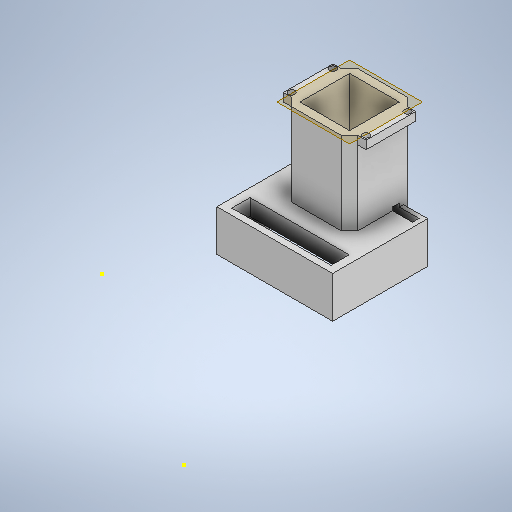
# Autodesk Inventor part: Soporte camara
Saved by Autodesk Inventor 2025 (Build 290162000, 162)
## iProperties
Created: 2025-02-01
Part Number: Soporte camara
Material: Genérico
Document SubType Name: Modeling
Designer: Jorge
Density: 1 g/cm^3
Appearance: Valor por defecto
Author: Jorge
Autodesk Inventor part; units mm, degrees
ref_plane "YZ Plane" through (0, 0, 0) normal (1, 0, 0) x (0, 1, 0)
sketch "Boceto1" plane through (0, 0, 0) normal (0, 1, 0) x (-1, 0, 0)
  line L0 (0, 0) -> (0, -154)
  line L1 (35, -185) -> (95, -185)
  line L2 (130, -154) -> (130, 0)
  line L3 (130, 0) -> (0, 0)
  line L4 (0, 0) -> (0, -154) construction
  line L5 (65, -185) -> (95, -185) construction
  line L6 (95, -185) -> (95, -206.4869) construction
  line L7 (95, -206.4869) -> (35, -206.4869) construction
  line L8 (35, -206.4869) -> (35, -185) construction
  line L9 (0, -154) -> (35, -185)
  line L10 (95, -185) -> (130, -154)
  line L11 (61.4516, 0) -> (61.4516, -5) construction
  line L12 (130, -81.3037) -> (125, -81.3037) construction
  line L13 (0, -85.0807) -> (5, -85.0807) construction
  line L14 (125, -5) -> (5, -5)
  line L15 (5, -5) -> (5, -148.3548)
  line L16 (125, -148.3548) -> (125, -5)
  line L17 (112.5, -169.5) -> (109.1848, -165.7571) construction
  line L18 (65, -185) -> (65, -180) construction
  line L19 (17.5, -169.5) -> (20.8152, -165.7571) construction
  line L20 (20.8152, -165.7571) -> (5, -151.7493)
  line L21 (20.8152, -165.7571) -> (36.8959, -180)
  line L22 (36.8959, -180) -> (93.1041, -180)
  line L23 (93.1041, -180) -> (125, -151.7493)
  line L24 (125, -151.7493) -> (125, -148.3548)
  line L25 (5, -148.3548) -> (5, -151.7493)
  dimension "d2" = 154
  dimension "d3" = 30
  dimension "d4" = 60
  dimension "d5" = 5
  dimension "d6" = 5
  dimension "d7" = 5
  dimension "d8" = 5
  dimension "d9" = 5
  dimension "d10" = 5
  constraints: 52 end point, 9 perpendicular, 4 horizontal, 3 midpoint, 3 point on line, 3 vertical, 2 parallel
  measures "d2" distance of L0.end L0.start
  measures "d3" distance of L1.end L5.start
  measures "d4" distance of L6.end L7.end
  measures "d5" distance of L11.start L11.end
  measures "d6" distance of L12.start L12.end
  measures "d7" distance of L13.start L13.end
  measures "d8" distance of L17.start L17.end
  measures "d9" distance of L5.start L18.end
  measures "d10" distance of L19.start L19.end
extrude "Extrusión1" add sketch "Boceto1" along normal blind 3 contours L16 L24 L23 L22 L21 L20 L25 L15 L14
extrude "Extrusión2" add sketch "Boceto1" along normal blind 35
ref_plane "Plano de trabajo1" through (0, 20, 0) normal (0, 1, 0) x (-1, 0, 0)
sketch "Boceto2" plane through (0, 20, 0) normal (0, 1, 0) x (-1, 0, 0)
  line L0 (0, 0) -> (0, -154) construction
  line L1 (0, 0) -> (0, -26.749) construction
  line L2 (130, -154) -> (130, 0) construction
  line L3 (125, -151.7493) -> (93.1041, -180) construction
  line L4 (125, -151.7493) -> (5, -151.7493) construction
  line L5 (65, -151.7493) -> (65, -26.749) construction
  line L6 (125, -89.2492) -> (5, -89.2492) construction
  line L7 (5, -151.7493) -> (5, -5) construction
  line L8 (125, -26.749) -> (125, -31.749) construction
  line L9 (125, -31.749) -> (120, -31.749) construction
  line L10 (120, -31.749) -> (120, -26.749) construction
  line L11 (125, -31.749) -> (120, -26.749) construction
  line L12 (120, -31.749) -> (125, -26.749) construction
  line L13 (125, -31.749) -> (125, -26.749)
  arc A0 (120, -26.749) -> (125, -31.749) centre (122.5, -29.249) ccw
  line L14 (5, -26.749) -> (5, -31.749) construction
  line L15 (5, -31.749) -> (5, -26.749)
  arc A1 (5, -31.749) -> (10, -26.749) centre (7.5, -29.249) ccw
  arc A2 (125, -26.749) -> (120.5, -32.1645) centre (122.5, -29.249) ccw
  arc A3 (10.6306, -27.606) -> (5, -26.749) centre (7.5, -29.249) ccw
  line L16 (5, -26.749) -> (5, -173.4983) construction
  line L17 (125, -151.7493) -> (125, -146.7493) construction
  line L18 (120, -146.7493) -> (125, -151.7493) construction
  line L19 (125, -146.7493) -> (125, -151.7493)
  arc A4 (125, -146.7493) -> (120, -151.7493) centre (122.5, -149.2493) ccw
  arc A5 (10, -151.7493) -> (5, -146.7493) centre (7.5, -149.2493) ccw
  line L20 (5, -151.7493) -> (5, -146.7493) construction
  line L21 (5, -146.7493) -> (5, -151.7493)
  arc A6 (120.5, -146.3339) -> (125, -151.7493) centre (122.5, -149.2493) ccw
  arc A7 (5, -151.7493) -> (10.6306, -150.8923) centre (7.5, -149.2493) ccw
  circle A8 centre (7.5, -29.249) radius 2.5
  circle A9 centre (122.5, -29.249) radius 2.5
  circle A10 centre (122.5, -149.2493) radius 2.5
  circle A11 centre (7.5, -149.2493) radius 2.5
  point P0 (10, -151.7493)
  point P1 (10, -26.749)
  point P2 (120, -26.749)
  dimension "d16" = 26.749
  dimension "d43" = 5
  dimension "d44" = 5
  dimension "d45" = 5
  dimension "d46" = 5
  constraints: 36 end point, 20 point on circle, 18 symmetric about line, 12 centre point, 5 coincident, 2 perpendicular, 2 point on line, 1 horizontal, 1 midpoint, 5 other
  measures "d16" distance of L0.start L1.end
  measures "d43" diameter of A8
  measures "d44" diameter of A9
  measures "d45" diameter of A10
  measures "d46" diameter of A11
extrude "Extrusión3" add sketch "Boceto2" against normal blind 17 contours A9 | A0 A2 L13 | A8 | L15 A3 A1 | A10 | L19 A6 A4 | A11 | A7 L21 A5
extrude "Extrusión4" cut sketch "Boceto2" against normal through all contours A9 | A8 | A10 | A11
sketch "Boceto3" plane through (0, 3, 0) normal (0, 1, 0) x (1, 0, 0)
  line L0 (-125, 5) -> (-5, 5) construction
  line L1 (-65, 5) -> (-110, 5) construction
  line L2 (-110, 5) -> (-110, 15) construction
  line L3 (-110, 15) -> (-20, 15)
  line L4 (-20, 15) -> (-20, 139.5644)
  line L5 (-110, 139.5644) -> (-110, 15)
  line L6 (-106.9205, 15) -> (-103.9205, 15)
  line L7 (-20, 139.5644) -> (-20, 15)
  line L8 (-110, 15) -> (-20, 15)
  line L9 (-110, 15) -> (-110, 139.5644)
  line L10 (-83.4405, 15) -> (-81.4405, 15)
  line L11 (-77.5705, 15) -> (-75.5705, 15)
  line L12 (-87.3105, 15) -> (-89.3105, 15)
  line L13 (-93.1805, 15) -> (-95.1805, 15)
  line L14 (-98.0505, 15) -> (-100.0505, 15)
  line L15 (-103.9205, 15) -> (-106.9205, 15)
  line L16 (-71.7005, 15) -> (-69.7005, 15)
  line L17 (-65.8305, 15) -> (-63.8305, 15)
  line L18 (-59.9605, 15) -> (-57.9605, 15)
  line L19 (-54.0905, 15) -> (-52.0905, 15)
  line L20 (-48.2205, 15) -> (-46.2205, 15)
  line L21 (-42.3505, 15) -> (-40.3505, 15)
  line L22 (-36.4805, 15) -> (-34.4805, 15)
  line L23 (-30.6105, 15) -> (-28.6105, 15)
  line L24 (-24.7405, 15) -> (-22.7405, 15)
  line L25 (-35, 185) -> (-95, 185) projected
  line L26 (-20, 139.5644) -> (-110, 139.5644)
  line L27 (-103.9205, 15) -> (-103.9205, 139.5644)
  line L28 (-106.9205, 139.5644) -> (-106.9205, 15)
  line L29 (-100.9205, 15) -> (-100.9205, 139.5644)
  line L30 (-103.9205, 139.5644) -> (-103.9205, 15)
  line L31 (-97.9205, 15) -> (-97.9205, 139.5644)
  line L32 (-100.9205, 139.5644) -> (-100.9205, 15)
  line L33 (-94.9205, 15) -> (-94.9205, 139.5644)
  line L34 (-97.9205, 139.5644) -> (-97.9205, 15)
  line L35 (-91.9205, 15) -> (-91.9205, 139.5644)
  line L36 (-94.9205, 139.5644) -> (-94.9205, 15)
  line L37 (-88.9205, 15) -> (-88.9205, 139.5644)
  line L38 (-91.9205, 139.5644) -> (-91.9205, 15)
  line L39 (-85.9205, 15) -> (-85.9205, 139.5644)
  line L40 (-88.9205, 139.5644) -> (-88.9205, 15)
  line L41 (-82.9205, 15) -> (-82.9205, 139.5644)
  line L42 (-85.9205, 139.5644) -> (-85.9205, 15)
  line L43 (-79.9205, 15) -> (-79.9205, 139.5644)
  line L44 (-82.9205, 139.5644) -> (-82.9205, 15)
  line L45 (-76.9205, 15) -> (-76.9205, 139.5644)
  line L46 (-79.9205, 139.5644) -> (-79.9205, 15)
  line L47 (-73.9205, 15) -> (-73.9205, 139.5644)
  line L48 (-76.9205, 139.5644) -> (-76.9205, 15)
  line L49 (-70.9205, 15) -> (-70.9205, 139.5644)
  line L50 (-73.9205, 139.5644) -> (-73.9205, 15)
  line L51 (-67.9205, 15) -> (-67.9205, 139.5644)
  line L52 (-70.9205, 139.5644) -> (-70.9205, 15)
  line L53 (-64.9205, 15) -> (-64.9205, 139.5644)
  line L54 (-67.9205, 139.5644) -> (-67.9205, 15)
  line L55 (-61.9205, 15) -> (-61.9205, 139.5644)
  line L56 (-64.9205, 139.5644) -> (-64.9205, 15)
  line L57 (-58.9205, 15) -> (-58.9205, 139.5644)
  line L58 (-61.9205, 139.5644) -> (-61.9205, 15)
  line L59 (-55.9205, 15) -> (-55.9205, 139.5644)
  line L60 (-58.9205, 139.5644) -> (-58.9205, 15)
  line L61 (-52.9205, 15) -> (-52.9205, 139.5644)
  line L62 (-55.9205, 139.5644) -> (-55.9205, 15)
  line L63 (-49.9205, 15) -> (-49.9205, 139.5644)
  line L64 (-52.9205, 139.5644) -> (-52.9205, 15)
  line L65 (-46.9205, 15) -> (-46.9205, 139.5644)
  line L66 (-49.9205, 139.5644) -> (-49.9205, 15)
  line L67 (-43.9205, 15) -> (-43.9205, 139.5644)
  line L68 (-46.9205, 139.5644) -> (-46.9205, 15)
  line L69 (-40.9205, 15) -> (-40.9205, 139.5644)
  line L70 (-43.9205, 139.5644) -> (-43.9205, 15)
  line L71 (-37.9205, 15) -> (-37.9205, 139.5644)
  line L72 (-40.9205, 139.5644) -> (-40.9205, 15)
  line L73 (-34.9205, 15) -> (-34.9205, 139.5644)
  line L74 (-37.9205, 139.5644) -> (-37.9205, 15)
  line L75 (-31.9205, 15) -> (-31.9205, 139.5644)
  line L76 (-34.9205, 139.5644) -> (-34.9205, 15)
  line L77 (-28.9205, 15) -> (-28.9205, 139.5644)
  line L78 (-31.9205, 139.5644) -> (-31.9205, 15)
  line L79 (-25.9205, 15) -> (-25.9205, 139.5644)
  line L80 (-28.9205, 139.5644) -> (-28.9205, 15)
  line L81 (-22.9205, 15) -> (-22.9205, 139.5644)
  line L82 (-25.9205, 139.5644) -> (-25.9205, 15)
  point P0 (0, 0)
  dimension "d24" = 45
  dimension "d25" = 10
  dimension "d32" = 5.87
  dimension "d47" = 3
  dimension "d50" = 3
  constraints: 158 end point, 108 horizontal alignment, 57 parallel, 9 horizontal, 7 collinear, 3 vertical, 2 perpendicular, 1 midpoint, 1 point on line, 9 other
  measures "d24" distance of L1.start L1.end
  measures "d25" distance of L1.end L2.end
  measures "d32" distance of L6.end L14.start
  measures "d47" distance between parallel lines of L27 L28
  measures "d50" distance of L6.end L29.start
extrude "Extrusión5" cut sketch "Boceto3" against normal blind 10 contours L5 L26 L28 L3 | L27 L26 L29 L3 | L26 L33 L3 L31 | L26 L37 L3 L35 | L26 L41 L3 L39 | L26 L45 L3 L43 | L26 L49 L3 L47 | L26 L53 L3 L51 | L26 L57 L3 L55 | L26 L61 L3 L59 | L26 L65 L3 L63 | L26 L69 L3 L67 | L26 L73 L3 L71 | L26 L77 L3 L75 | L26 L81 L3 L79
fillet "Empalme1" radius 5 4 edges at (-130, 17.5, 0) (0, 17.5, 0) (0, 17.5, -154) (-130, 17.5, -154)
fillet "Empalme2" radius 5 2 edges at (-95, 17.5, -185) (-35, 17.5, -185)
sketch "Sketch5" plane through (-125, 3, -146.7493) normal (1, 0, 0) x (0, 0, -1)
  line L0 (0, 0) -> (-115.0003, 0) construction
  line L1 (-110.8969, 0) -> (-110.8969, 17.0593) construction
  line L2 (-4.4814, 0) -> (-4.4814, 32) construction
  line L3 (-141.7493, 32) -> (5, 32) construction
  line L4 (-110.8969, 0) -> (-4.4814, 0)
  line L5 (-4.4814, 0) -> (-4.4814, 25.5232)
  line L6 (-4.4814, 25.5232) -> (-110.8969, 25.5232)
  line L7 (-110.8969, 25.5232) -> (-110.8969, 0)
  line L8 (-110.8969, 25.5232) -> (-4.4814, 25.5232)
  line L9 (-4.4814, 25.5232) -> (-4.4814, 52.7113)
  line L10 (-4.4814, 52.7113) -> (-110.8969, 52.7113)
  line L11 (-110.8969, 52.7113) -> (-110.8969, 25.5232)
  point P0 (-146.7493, -3)
  point P1 (-115.0003, 17)
  point P2 (0, 17)
  point P3 (5, 32)
  constraints: 20 end point, 4 parallel, 2 horizontal, 2 perpendicular, 2 point on line, 2 vertical, 2 other
extrude "Extrusion6" cut sketch "Sketch5" against normal through all
sketch "Sketch6" plane through (-122.5, 20, -29.249) normal (0, 1, 0) x (1, 0, 0)
  arc A0 (-2.5, -2.5) -> (-2.5, 2.5) centre (0, 0) ccw projected
  circle A1 centre (0, 0) radius 2.5 projected
  arc A2 (-2.5, 117.5003) -> (-2.1798, 122.784) centre (0, 120.0003) ccw projected
  circle A3 centre (0, 120.0003) radius 2.5 projected
  arc A4 (117.1798, 122.784) -> (117.5, 117.5003) centre (115, 120.0003) ccw projected
  circle A5 centre (115, 120.0003) radius 2.5 projected
  circle A6 centre (115, 0) radius 2.5 projected
  arc A7 (117.5, 2.5) -> (117.5, -2.5) centre (115, 0) ccw projected
  circle A8 centre (0, 0) radius 2.5
  circle A9 centre (0, 0) radius 3.5355
  circle A10 centre (0, 120.0003) radius 2.5
  circle A11 centre (0, 120.0003) radius 3.5355
  circle A12 centre (115, 120.0003) radius 2.5
  circle A13 centre (115, 120.0003) radius 3.5355
  circle A14 centre (115, 0) radius 2.5
  circle A15 centre (115, 0) radius 3.5355
  point P0 (122.5, -29.249)
  point P1 (-2.5, 0)
  point P2 (-2.5, 120.0003)
  point P3 (117.5, 120.0003)
  point P4 (117.5, 0)
  point P5 (-2.5, -2.5)
  point P6 (-2.5, 117.5003)
  point P7 (117.5, 117.5003)
  point P8 (117.5, -2.5)
  constraints: 8 centre point, 8 coincident, 4 concentric, 4 horizontal alignment, 4 other
extrude "Extrusion7" add sketch "Sketch6" along normal blind 15
sketch "Sketch7" plane through (0, 0, 0) normal (0, -1, 0) x (1, 0, 0)
  line L0 (-36.8959, -185) -> (-93.1041, -185) construction
  line L1 (-65, -185) -> (-65, 0) construction
  line L2 (-125, 0) -> (-5, 0) construction
  line L3 (-130, -35.8525) -> (-130, -142.2679) construction
  line L4 (-130, -142.2679) -> (0, -142.2679) construction
  line L5 (-65, -185) -> (-85, -185) construction
  line L6 (-65, -185) -> (-45, -185) construction
  line L7 (-45, -185) -> (-45, -145) construction
  line L8 (-45, -145) -> (-85, -145) construction
  line L9 (-45, -145) -> (-85, -145)
  line L10 (-85, -145) -> (-85, -185)
  line L11 (-85, -185) -> (-45, -185)
  line L12 (-45, -185) -> (-45, -145)
  point P0 (0, 0)
  dimension "d57" = 20
  dimension "d58" = 20
  dimension "d59" = 40
  constraints: 20 end point, 3 parallel, 3 perpendicular, 2 midpoint, 2 point on line, 1 horizontal
  measures "d57" distance of L1.start L5.end
  measures "d58" distance of L1.start L6.end
  measures "d59" distance of L6.end L7.end
extrude "Extrusion8" add sketch "Sketch7" along normal blind 50
sketch "Sketch8" plane through (0, -50, 0) normal (0, -1, 0) x (1, 0, 0)
  line L0 (-45, -185) -> (-45, -145) construction
  line L1 (-45, -145) -> (-85.5281, -185) construction
  line L2 (-36.8959, -185) -> (-93.1041, -185) construction
  line L3 (-85, -145) -> (-85, -185) construction
  line L4 (-85, -145) -> (-45.5212, -185) construction
  line L5 (-32.7606, -175) -> (-32.7606, -137.5)
  line L6 (-32.7606, -137.5) -> (-97.7606, -137.5)
  line L7 (-97.7606, -137.5) -> (-97.7606, -175)
  line L8 (-97.7606, -192.5) -> (-32.7606, -137.5) construction
  line L9 (-32.7606, -192.5) -> (-97.7606, -137.5) construction
  line L10 (-30.2606, -195) -> (-100.2606, -195)
  line L11 (-100.2606, -195) -> (-100.2606, -135)
  line L12 (-100.2606, -135) -> (-30.2606, -195) construction
  line L13 (-30.2606, -135) -> (-100.2606, -195) construction
  line L14 (-65.2606, -135) -> (-65.2606, -130) construction
  line L15 (-65.2606, -130) -> (-100.2606, -130)
  line L16 (-100.2606, -130) -> (-100.2606, -135)
  line L17 (-30.2606, -135) -> (-30.2606, -130)
  line L18 (-30.2606, -130) -> (-65.2606, -130)
  line L19 (-65.2606, -130) -> (-65.2606, -125) construction
  line L20 (-64.9205, -139.5644) -> (-64.9205, -15) construction
  line L21 (-65.2606, -125) -> (-100.2606, -125)
  line L22 (-100.9205, -139.5644) -> (-100.9205, -15) projected
  line L23 (-100.2606, -130) -> (-100.2606, -125)
  line L24 (-65.2606, -125) -> (-30.2606, -125)
  line L25 (-30.2606, -125) -> (-30.2606, -130)
  line L26 (-65.2606, -125) -> (-65.2606, -120) construction
  line L27 (-100.2606, -125) -> (-100.2606, -120)
  line L28 (-100.2606, -120) -> (-65.2606, -120)
  line L29 (-65.2606, -120) -> (-30.2606, -120)
  line L30 (-30.2606, -120) -> (-30.2606, -125)
  line L31 (-100.2606, -195) -> (-100.2606, -175) construction
  line L32 (-97.7606, -175) -> (-32.7606, -175)
  line L33 (-97.7606, -192.5) -> (-97.3439, -192.5)
  line L34 (-33.1773, -192.5) -> (-32.7606, -192.5)
  line L35 (-32.7606, -175) -> (-32.7606, -177.5) construction
  line L36 (-30.2606, -177.5) -> (-100.2606, -177.5)
  line L37 (-30.2606, -135) -> (-30.2606, -195)
  line L38 (-28.9205, -15) -> (-28.9205, -139.5644) projected
  point P0 (0, 0)
  point P1 (-65.2606, -165)
  point P2 (-64.9205, -15)
  dimension "d62" = 65
  dimension "d63" = 55
  dimension "d64" = 70
  dimension "d65" = 60
  dimension "d96" = 5
  dimension "d101" = 5
  dimension "d112" = 20
  dimension "d113" = 2.5
  constraints: 66 end point, 8 perpendicular, 8 point on line, 5 midpoint, 4 parallel, 4 vertical, 3 horizontal, 2 collinear, 1 other
  measures "d62" distance of L6.end L5.end
  measures "d63" distance of L5.end L9.start
  measures "d64" distance of L10.start L10.end
  measures "d65" distance of L13.start L10.start
  measures "d96" distance of L14.end L19.end
  measures "d101" distance of L19.end L26.end
  measures "d112" distance of L10.end L31.end
  measures "d113" distance of L5.start L35.end
extrude "Extrusion9" add sketch "Sketch8" along normal blind 10 contours L32 L7 L6 L5
extrude "Extrusion10" add sketch "Sketch8" along normal blind 25 contours L18 L15 L23 L21 L24 L25 | L24 L21 L27 L28 L29 L30
chamfer "Chamfer3" distance 5 angle 45 2 edges at (-85, -25, -145) (-45, -25, -145)
ref_plane "Work Plane2" through (0, -75, 0) normal (0, -1, 0) x (1, 0, 0)
chamfer "Chamfer4" distance 5 angle 45 2 edges at (-45, -25, -185) (-85, -25, -185)
sketch "Sketch12" plane through (0, -75, 0) normal (0, -1, 0) x (1, 0, 0)
  point P0 (0, 0)
sketch "Sketch13" plane through (0, -75, 0) normal (0, -1, 0) x (1, 0, 0)
  line L0 (-30.2606, -125) -> (-100.2606, -125) construction
  line L1 (-97.7606, -137.5) -> (-32.7606, -137.5) construction
  line L2 (-65.2606, -137.5) -> (-65.2606, -125) construction
  line L3 (-97.7606, -137.5) -> (-97.7606, -125) construction
  line L4 (-32.7606, -137.5) -> (-32.7606, -125) construction
  line L5 (-97.7606, -131.25) -> (-32.7606, -131.25) construction
  line L6 (-95.2606, -136.25) -> (-35.2606, -126.25) construction
  line L7 (-35.2606, -136.25) -> (-95.2606, -126.25) construction
  line L8 (-30.2606, -120) -> (-100.2606, -120) construction
  line L9 (-97.7606, -125) -> (-97.9205, -120) construction
  line L10 (-97.9205, -15) -> (-97.9205, -139.5644) construction
  line L11 (-35.2606, -126.25) -> (-35.2606, -120) construction
  line L12 (-32.7606, -137.5) -> (-32.7606, -192.5) construction
  line L13 (-97.7606, -120) -> (-32.7606, -137.5) construction
  line L14 (-97.7606, -137.5) -> (-31.9205, -120) construction
  line L15 (-31.9205, -15) -> (-31.9205, -139.5644) construction
  line L16 (-95.0519, -133.8062) -> (-35.0519, -133.8062)
  line L17 (-35.0519, -133.8062) -> (-35.0519, -123.8062)
  line L18 (-35.0519, -123.8062) -> (-95.0519, -123.8062)
  line L19 (-95.0519, -123.8062) -> (-95.0519, -133.8062)
  line L20 (-95.0519, -133.8062) -> (-35.0519, -123.8062) construction
  line L21 (-35.0519, -133.8062) -> (-95.0519, -123.8062) construction
  point P0 (0, 0)
  point P1 (-65.2606, -131.25)
  point P2 (-65.0519, -128.8062)
  dimension "d102" = 60
  dimension "d103" = 10
  constraints: 32 end point, 10 point on line, 9 midpoint, 4 perpendicular, 2 parallel, 1 horizontal
  measures "d102" distance of L18.end L17.end
  measures "d103" distance of L17.end L16.end
extrude "Extrusion12" cut sketch "Sketch13" against normal blind 25
sketch "Sketch14" plane through (0, -75, 0) normal (0, -1, 0) x (1, 0, 0)
  line L0 (-32.7606, -137.5) -> (-32.7606, -192.5) projected
  line L1 (-95.0519, -130) -> (-95.0519, -123.8062) projected
  line L2 (-95.0519, -123.8062) -> (-35.0519, -123.8062) projected
  line L3 (-97.7606, -192.5) -> (-97.7606, -137.5) projected
  line L4 (-32.7606, -137.5) -> (-97.7606, -137.5)
  line L5 (-97.7606, -137.5) -> (-97.7606, -123.8062)
  line L6 (-97.7606, -123.8062) -> (-32.7606, -123.8062)
  line L7 (-32.7606, -123.8062) -> (-32.7606, -137.5)
  point P0 (0, 0)
  point P1 (-95.0519, -133.8062)
  constraints: 8 end point, 2 parallel, 1 horizontal, 1 perpendicular
extrude "Extrusion13" cut sketch "Sketch14" against normal blind 15
sketch "Sketch16" plane through (0, -60, 0) normal (0, -1, 0) x (1, 0, 0)
  line L0 (-85, -150) -> (-85, -175) projected
  line L1 (-85, -150) -> (-80, -145) projected
  line L2 (-50, -145) -> (-80, -145) projected
  line L3 (-50, -145) -> (-45, -150) projected
  line L4 (-45, -175) -> (-45, -150) projected
  line L5 (-45, -180) -> (-50, -185) projected
  line L6 (-80, -185) -> (-50, -185) projected
  line L7 (-80, -185) -> (-85, -180) projected
  line L8 (-50, -150) -> (-80, -150)
  line L9 (-80, -150) -> (-80, -180)
  line L10 (-80, -180) -> (-50, -180)
  line L11 (-50, -180) -> (-50, -150)
  line L12 (-50, -150) -> (-80, -180) construction
  line L13 (-80, -150) -> (-50, -180) construction
  point P0 (0, 0)
  point P1 (-65, -165)
  dimension "d108" = 30
  dimension "d109" = 30
  constraints: 12 end point, 2 midpoint, 2 parallel, 1 horizontal, 1 perpendicular
  measures "d108" distance of L10.end L9.end
  measures "d109" distance of L9.end L8.end
extrude "Extrusion15" cut sketch "Sketch16" against normal blind 60
sketch "Sketch17" plane through (-50, -60, -180) normal (-1, 0, 0) x (0, 0, 1)
  line L0 (30, 0) -> (5, 0) projected
  point P0 (180, 60)
  point P1 (0, 0)
extrude "Extrusion16" add sketch "Sketch8" along normal blind 25 contours L36 L11 L16 L15 L18 L17 L37
sketch "Sketch18" plane through (-50, -50, -177.5) normal (0, 0, -1) x (-1, 0, 0)
  line L0 (47.7606, -10) -> (47.7606, -25) projected
  line L1 (-17.2394, -10) -> (-17.2394, -25) projected
  line L2 (47.7606, -10) -> (-17.2394, -10)
  line L3 (-19.7394, 0) -> (-19.7394, -25) projected
  line L4 (-17.2394, -25) -> (-17.2394, -35.5392)
  line L5 (-17.2394, -35.5392) -> (47.7606, -35.5392)
  line L6 (47.7606, -35.5392) -> (47.7606, -25)
  point P0 (-50, 50)
  constraints: 8 end point, 3 perpendicular, 1 vertical
extrude "Extrusion17" cut sketch "Sketch18" against normal blind 47.75
sketch "Sketch19" plane through (0, -50, 0) normal (0, -1, 0) x (1, 0, 0)
  line L0 (-80, -185) -> (-50, -185) projected
  line L1 (-80, -185) -> (-85, -180) projected
  line L2 (-85, -177.5) -> (-85, -180) projected
  line L3 (-80, -180) -> (-80, -177.5) projected
  line L4 (-50, -180) -> (-80, -180) projected
  line L5 (-50, -177.5) -> (-50, -180) projected
  line L6 (-45, -180) -> (-45, -177.5) projected
  line L7 (-45, -180) -> (-50, -185) projected
  line L8 (-45, -177.5) -> (-50, -177.5) projected
  line L9 (-80, -177.5) -> (-85, -177.5) projected
  line L10 (-80, -177.5) -> (-50, -177.5) projected
  line L11 (-50, -177.5) -> (-80, -177.5)
  point P0 (0, 0)
  constraints: 2 end point, 1 horizontal
extrude "Extrusion18" add sketch "Sketch19" along normal blind 10
sketch "Sketch20" plane through (0, 0, 0) normal (0, -1, 0) x (1, 0, 0)
  line L0 (-85, -180) -> (-80, -185) projected
  line L1 (-80, -185) -> (-85, -180)
  line L2 (-80, -145) -> (-85, -150) projected
  line L3 (-85, -180) -> (-85, -150)
  line L4 (-85, -150) -> (-80, -145)
  line L5 (-80, -145) -> (-49.9656, -145)
  line L6 (-93.1041, -180) -> (-36.8959, -180) projected
  line L7 (-49.9656, -145) -> (-44.9656, -150)
  line L8 (-44.9656, -150) -> (-44.9656, -180)
  line L9 (-36.8959, -185) -> (-93.1041, -185) projected
  line L10 (-44.9656, -180) -> (-49.9656, -185)
  line L11 (-36.8959, -185) -> (-50, -185) projected
  line L12 (-49.9656, -185) -> (-36.8959, -185)
  line L13 (-36.8959, -185) -> (24.1886, -177.7709)
  line L14 (24.1886, -177.7709) -> (33.2133, -87.4202)
  line L15 (33.2133, -87.4202) -> (33.6029, -83.52)
  line L16 (33.6029, -83.52) -> (59.5118, 20.6859)
  arc A0 (54.7558, 22.225) -> (59.5118, 20.6859) centre (68.223, 55.7226) ccw
  line L17 (54.7558, 22.225) -> (-146.3613, 43.1407)
  arc A1 (-146.3613, 43.1407) -> (-154.6578, 39.9856) centre (-147.3809, 33.3364) ccw
  line L18 (-154.6578, 39.9856) -> (-200.8291, -46.8166)
  line L19 (-200.8291, -46.8166) -> (-163.556, -203.1842)
  line L20 (-163.556, -203.1842) -> (-92.4425, -201.8425)
  line L21 (-92.4425, -201.8425) -> (-85, -194.4)
  line L22 (-85, -194.4) -> (-80, -185)
  line L23 (-85, -180) -> (-85, -150)
  point P0 (0, 0)
  constraints: 38 end point, 5 parallel, 4 point on circle, 3 collinear, 3 point on line, 2 centre point, 1 perpendicular, 1 tangent, 1 vertical
extrude "Extrusion19" cut sketch "Sketch20" against normal through all contours L0 L22 L21 L20 L19 L18 A1 L17 A0 L16 L15 L14 L13 L9 L10 L8 L7 L5 L2 L3
sketch "Sketch21" plane through (-50, -60, -185) normal (0, 0, -1) x (-1, 0, 0)
  line L0 (-5, 10) -> (-5, 60) projected
  line L1 (-5, 60) -> (49.1313, 60)
  line L2 (30, 60) -> (0, 60) projected
  line L3 (49.1313, 60) -> (53.9419, 116.0083)
  arc A0 (25.0787, 120.8189) -> (53.9419, 116.0083) centre (69.7131, 299.6306) ccw
  line L4 (25.0787, 120.8189) -> (-113.7396, 139.0302)
  arc A1 (-113.7396, 139.0302) -> (-109.2726, 107.0745) centre (-53.6227, 131.1436) ccw
  line L5 (-109.2726, 107.0745) -> (-56.0721, 40.422)
  line L6 (-56.0721, 40.422) -> (-11.9959, 40.422)
  line L7 (-11.9959, 40.422) -> (-11.9959, 60)
  line L8 (-11.9959, 60) -> (-5, 60)
  point P0 (-50, 60)
  constraints: 14 end point, 4 point on circle, 3 point on line, 2 centre point, 2 perpendicular, 1 collinear
extrude "Extrusion20" cut sketch "Sketch21" against normal through all
ref_plane "Work Plane3" through (-80, 0, -185) normal (0, 1, 0) x (1, 0, 0)
sketch "Sketch23" plane through (-80, 0, -185) normal (0, 1, 0) x (1, 0, 0)
  line L0 (-5, -5) -> (-10, -5)
  line L1 (-10, -5) -> (-10, -10)
  line L2 (-10, -10) -> (-5, -10)
  line L3 (-5, -10) -> (-5, -5)
  line L4 (-5, -35) -> (-5, -5) construction
  line L5 (-5, -20) -> (-15.783, -20) construction
  circle A0 centre (-7.5, -7.5) radius 2
  line L6 (-5, -35) -> (-10, -35)
  line L7 (-10, -35) -> (-10, -30)
  line L8 (-10, -30) -> (-5, -30)
  line L9 (-5, -30) -> (-5, -35)
  circle A1 centre (-7.5, -32.5) radius 2
  line L10 (35, -35) -> (35, -5) construction
  line L11 (35, -5) -> (40, -5)
  line L12 (40, -5) -> (40, -10)
  line L13 (40, -10) -> (35, -10)
  line L14 (35, -10) -> (35, -5)
  circle A2 centre (37.5, -7.5) radius 2
  line L15 (35, -20) -> (51.9517, -20) construction
  line L16 (35, -5) -> (35, -35) construction
  line L17 (35, -35) -> (40, -35)
  line L18 (40, -35) -> (40, -30)
  line L19 (40, -30) -> (35, -30)
  line L20 (35, -30) -> (35, -35)
  circle A3 centre (37.5, -32.5) radius 2
  point P0 (80, -185)
  dimension "d125" = 5
  dimension "d126" = 5
  dimension "d127" = 4
  dimension "d128" = 5
  dimension "d129" = 5
  dimension "d130" = 4
  constraints: 38 end point, 10 symmetric about line, 4 centre point, 4 horizontal, 4 parallel, 2 midpoint, 2 perpendicular, 2 other
  measures "d125" distance of L2.end L1.end
  measures "d126" distance of L1.end L0.end
  measures "d127" diameter of A0
  measures "d128" distance of L12.end L13.end
  measures "d129" distance of L11.end L12.end
  measures "d130" diameter of A2
extrude "Extrusion21" add sketch "Sketch23" against normal blind 5
sketch "Sketch24" plane through (-45, 0, -175) normal (0, 0, 1) x (1, 0, 0)
  line L0 (0, -5) -> (0, 0) projected
  line L1 (5, -5) -> (0, -5) projected
  line L2 (0, 0) -> (5, 0) projected
  line L3 (0, -5) -> (0, 0) projected
  line L4 (5, -5) -> (0, -5) projected
  line L5 (5, 0) -> (5, -5) projected
  point P0 (45, 0)
extrude "Extrusion22" add sketch "Sketch24" along normal blind 20
sketch "Sketch25" plane through (-90, 0, -175) normal (0, 0, 1) x (1, 0, 0)
  line L0 (0, 0) -> (5, 0) projected
  line L1 (0, 0) -> (0, -5) projected
  line L2 (5, -5) -> (0, -5) projected
  line L3 (5, 0) -> (5, -5) projected
  point P0 (90, 0)
extrude "Extrusion23" add sketch "Sketch25" along normal blind 20
sketch "Sketch26" plane through (0, -60, 0) normal (0, -1, 0) x (1, 0, 0)
  line L0 (-80, -175) -> (-50, -175) projected
  line L1 (-80, -175) -> (-80, -150) projected
  line L2 (-50, -150) -> (-50, -175) projected
  line L3 (-32.7606, -177.5) -> (-32.7606, -123.8062) projected
  line L4 (-50, -175) -> (-50, -171) construction
  line L5 (-65, -175) -> (-33, -175) construction
  line L6 (-65, -175) -> (-96.8928, -172.3826) construction
  line L7 (-33, -175) -> (-97, -175)
  line L8 (-97, -175) -> (-97, -171)
  line L9 (-97, -171) -> (-33, -171)
  line L10 (-33, -171) -> (-33, -175)
  line L11 (-50, -171) -> (-80, -171)
  line L12 (-80, -171) -> (-80, -150)
  line L13 (-80, -150) -> (-50, -150)
  line L14 (-50, -150) -> (-50, -171)
  point P0 (0, 0)
  dimension "d137" = 4
  dimension "d138" = 32
  dimension "d139" = 32
  dimension "d140" = 64
  constraints: 22 end point, 4 parallel, 2 horizontal, 2 perpendicular, 2 point on line, 1 midpoint
  measures "d137" distance of L2.end L4.end
  measures "d138" distance of L5.start L5.end
  measures "d139" distance of L5.start L6.end
  measures "d140" distance of L8.end L9.end
extrude "Extrusion24" add sketch "Sketch26" against normal blind 6.75 contours L1 L13 L2 L9
extrude "Extrusion25" cut sketch "Sketch26" against normal blind 12 contours L7 L8 L9 L1 | L2 L9 L10 L7
sketch "Sketch27" plane through (0, -60, 0) normal (0, -1, 0) x (1, 0, 0)
  line L0 (-35.0519, -130) -> (-35.0519, -123.8062) projected
  line L1 (-35.0519, -123.8062) -> (-35.0519, -134.8062)
  line L2 (-95.0519, -123.8062) -> (-95.0519, -134.8062)
  line L3 (-95.0519, -134.8062) -> (-35.0519, -134.8062)
  line L4 (-35.0519, -130) -> (-38.8579, -126.9031)
  line L5 (-38.8579, -126.9031) -> (-80.7461, -125.972)
  line L6 (-80.7461, -125.972) -> (-93.5344, -126.9031)
  line L7 (-93.5344, -126.9031) -> (-95.0519, -130)
  point P0 (0, 0)
  dimension "d145" = 11
  dimension "d146" = 11
  constraints: 14 end point, 1 collinear, 1 point on line, 1 vertical
  measures "d145" distance of L0.end L1.end
  measures "d146" distance of L2.start L2.end
extrude "Extrusion26" cut sketch "Sketch27" against normal through all
